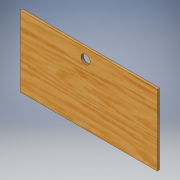
# Autodesk Inventor part: Devant - Bas Rammasse-Balle
Saved by Autodesk Inventor 2016 (Build 200138000, 138)
## iProperties
Created: 2016-01-24
Part Number: Devant - Bas Rammasse-Balle
Material: Generic
Document SubType Name: Modeling
Designer: ares-b02
Density: 1 g/cm^3
Appearance: Plywood - New
Author: ares-b02
Autodesk Inventor part; units mm, degrees
ref_plane "YZ Plane" through (0, 0, 0) normal (1, 0, 0) x (0, 1, 0)
ref_plane "XZ Plane" through (0, 0, 0) normal (0, 1, 0) x (-1, 0, 0)
ref_plane "XY Plane" through (0, 0, 0) normal (0, 0, 1) x (1, 0, 0)
sketch "Sketch1" plane through (0, 0, 0) normal (0, 0, 1) x (1, 0, 0)
  line L0 (-194.2621, 130.6481) -> (186.7379, 130.6481)
  line L1 (186.7379, 130.6481) -> (186.7379, -66.2019)
  line L2 (186.7379, -66.2019) -> (-194.2621, -66.2019)
  line L3 (-194.2621, -66.2019) -> (-194.2621, 130.6481)
  point P0 (0, 0)
  dimension "d0" = 381
  dimension "d1" = 196.85
  constraints: 8 end point, 2 parallel, 1 horizontal, 1 perpendicular
  measures "d0" distance of L0.start L0.end
  measures "d1" distance of L2.end L0.start
extrude "Extrusion1" add sketch "Sketch1" along normal blind 6.35
hole "Hole1" at (-12.7167, 103.2205, 6.35) direction (0, 0, -1) diameter 25.4 end through all
body "Solid1"
